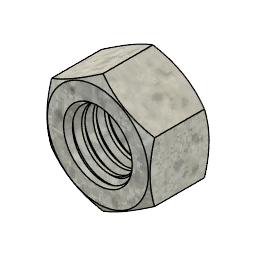
knob Foot (Autodesk Fusion 360 archive; units mm, degrees)
design "Hex Nut ASME B18.2.2 - 3/8-16 Steel Grade 2H Zinc"
description: Hex Nut ASME B18.2.2 - 3/8-16
part number: HN ASME B18.2.2 - 3/8-16 Steel Grade 2H Zinc
Autodesk Fusion 360 part; units mm, degrees
sketch "Sketch1" plane through (0, 0, 0) normal (0, 1, 0) x (1, 0, 0)
  line L0 (0, 0) -> (0, -8.3566)
  line L1 (-4.7625, 0) -> (-7.0071, 0)
  line L2 (-7.0071, 0) -> (-8.2584, -0.7224)
  line L3 (-8.2584, -0.7224) -> (-8.2584, -7.6342)
  line L4 (-8.2584, -7.6342) -> (-7.0071, -8.3566)
  line L5 (-7.0071, -8.3566) -> (-4.7625, -8.3566)
  line L6 (-4.7625, -8.3566) -> (-4.7625, 0)
  dimension "d121" = 9.525
  dimension "d122" = 30
  dimension "d123" = 30
  dimension "d128" = 16.5167
  dimension "d170" = 14.0142
  dimension "d176" = 8.3566
  constraint vertical L0
  constraint coincident L0 L0.end
  constraint coincident origin L0
  constraint horizontal L1
  constraint perpendicular L5 L6
  constraint coincident L0.start L1
  constraint coincident L0.end L5
  constraint coincident L0.start origin
  constraint vertical L1.end L4.end
  measures "d122" angle of L1 L2
  measures "d123" angle of L4 L5
  measures "d176" distance of L1.start L5
revolve "Revolve1" add sketch "Sketch1" angle 360 about axis through (0, 0, 0) along (0, 0, 1)
sketch "Sketch8" plane through (0, 0, 8.3566) normal (0, 0, 1) x (1, 0, 0)
  line L0 (-7.1501, -4.1324) -> (-7.1501, 4.1324)
  circle A0 centre (0, 0) radius 4.7625
  circle A1 centre (0, 0) radius 8.2584
  dimension "d114" = 7.1501
  constraint coincident L0.end A1
  constraint vertical L0
  constraint coincident L0.start A1
  measures "d114" distance of A0.centre L0
extrude "Extrude5" cut sketch "Sketch8" against normal blind 8.3566 contours L0 A1 picked at (-7.3289, -1.0065)
pattern_circular "C-Pattern2" count 6 over 360 about axis through (0, 0, 1.75) along (0, 0, 1) of "Extrude5"
thread "Thread3" "ANSI Unified Screw Threads 0.375 3/8-16 UNC 3/8-16 UNC 2B" major diameter 9.525 minor diameter 7.9756 pitch 1.5875 angle 60 modelled right hand crest width 0.4521 on face at (-4.7388, 0.4742, 5.5711) crest through (-3.9878, 0, 7.9597)
sketch "Sketch12" plane through (0, 0, 0) normal (0, 1, 0) x (1, 0, 0)
  line L0 (0, 0) -> (-4.7625, 0)
  line L1 (0, 0) -> (0, -8.3566)
  line L2 (0, -8.3566) -> (-4.7625, -8.3566)
  line L3 (-4.7625, -8.3566) -> (-2.3502, -4.1783)
  line L4 (-4.7625, 0) -> (-2.3502, -4.1783)
  dimension "d164" = 60
  dimension "d165" = 60
  dimension "d175" = 4.7625
  constraint coincident L0.start L1.start
  constraint horizontal L0
  constraint coincident L1.end L2.start
  constraint perpendicular L1 L2
  constraint vertical L0.end L2.end
  constraint coincident L3.end L4.end
  measures "d164" angle of L0 L4
  measures "d165" angle of L2 L3
  measures "d175" distance of L0.end L1
revolve "Revolve3" cut sketch "Sketch12" angle 360 about axis through (0, 0, 1.75) along (0, 0, 1)
equation "d89 = -adsk_nheig"
equation "d114 = adsk_waflat / 2"
equation "adsk_chamang1 = 30.00 deg"
equation "adsk_chamang2 = 30.00 deg"
equation "d121 = adsk_nomdia"
equation "d122 = adsk_chamang1"
equation "d123 = adsk_chamang2"
equation "d128 = adsk_maxdia"
equation "adsk_nheig = 0.329 in"
equation "adsk_maxdia = 0.650265 in"
equation "adsk_nomdia = 0.375 in"
equation "adsk_waflat = 0.563 in"
equation "d162 = adsk_nheig"
equation "adsk_beardia = adsk_waflat * 0.98"
equation "d170 = adsk_beardia"
equation "d175 = adsk_nomdia * 0.50"
equation "d176 = adsk_nheig"
